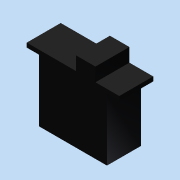
# Autodesk Inventor part: FUTABA-RS404PD Blank
Saved by Autodesk Inventor 2012 (Build 160160000, 160)
## iProperties
Created: 2012-05-22
Part Number: FUTABA-RS404PD Blank
Material: Default
Document SubType Name: Modeling
Designer: dgitz
Density: 1 g/cm^3
Author: dgitz
Autodesk Inventor part; units mm, degrees
ref_plane "YZ Plane" through (0, 0, 0) normal (1, 0, 0) x (0, 1, 0)
ref_plane "XZ Plane" through (0, 0, 0) normal (0, 1, 0) x (-1, 0, 0)
ref_plane "XY Plane" through (0, 0, 0) normal (0, 0, 1) x (1, 0, 0)
sketch "Sketch1" plane through (0, 0, 0) normal (0, 0, 1) x (1, 0, 0)
  line L0 (-69.1405, 36.1754) -> (-69.1405, 33.6354)
  line L1 (-69.1405, 33.6354) -> (-61.8905, 33.6354)
  line L2 (-61.8905, 33.6354) -> (-61.8905, -2.9246)
  line L3 (-61.8905, -2.9246) -> (-21.8905, -2.9246)
  line L4 (-21.8905, -2.9246) -> (-21.8905, 33.6354)
  line L5 (-21.8905, 33.6354) -> (-14.6405, 33.6354)
  line L6 (-14.6405, 33.6354) -> (-14.6405, 36.1754)
  line L7 (-14.6405, 36.1754) -> (-21.8905, 36.1754)
  line L8 (-21.8905, 36.1754) -> (-21.8905, 36.1754)
  line L9 (-21.8905, 36.1754) -> (-28.6829, 36.1754)
  line L10 (-28.6829, 36.1754) -> (-28.6829, 44.1754)
  line L11 (-28.6829, 44.1754) -> (-40.1582, 44.1754)
  line L12 (-40.1582, 44.1754) -> (-40.1582, 36.1754)
  line L13 (-40.1582, 36.1754) -> (-61.8905, 36.1754)
  line L14 (-61.8905, 36.1754) -> (-61.8905, 36.1754)
  line L15 (-61.8905, 36.1754) -> (-69.1405, 36.1754)
  dimension "d7" = 47.1
  dimension "d8" = 40
  dimension "d9" = 39.1
  dimension "d10" = 54.5
  dimension "d11" = 39.1
  dimension "d12" = 2.54
  constraints: 32 end point, 13 parallel, 4 collinear, 3 equal length, 1 perpendicular, 1 vertical
  measures "d7" distance between parallel lines of L11 L3
  measures "d8" distance between parallel lines of L4 L2
  measures "d9" distance between parallel lines of L15 L3
  measures "d10" distance between parallel lines of L6 L0
  measures "d11" distance between parallel lines of L13 L3
  measures "d12" distance between parallel lines of L15 L1
extrude "Extrusion1" add sketch "Sketch1" along normal mid plane 20
body "Solid1"
